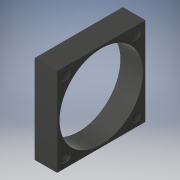
# Autodesk Inventor part: Pi Fan
Saved by Autodesk Inventor 2019 (Build 230136000, 136)
## iProperties
Created: 2018-04-04
Part Number: Pi Fan
Material: PPS Plastic
Document SubType Name: Modeling
Designer: Nikolas X Gamarra
Density: 1.637 g/cm^3
Appearance: Smooth - White(1)
Author: Nikolas X Gamarra
Autodesk Inventor part; units mm, degrees
ref_plane "YZ Plane" through (0, 0, 0) normal (1, 0, 0) x (0, 1, 0)
ref_plane "XZ Plane" through (0, 0, 0) normal (0, 1, 0) x (-1, 0, 0)
ref_plane "XY Plane" through (0, 0, 0) normal (0, 0, 1) x (1, 0, 0)
sketch "Sketch1" plane through (0, 0, 0) normal (1, 0, 0) x (0, 1, 0)
  line L0 (0, 0) -> (30, 0)
  line L1 (30, 0) -> (30, -30)
  line L2 (30, -30) -> (0, -30)
  line L3 (0, -30) -> (0, 0)
  dimension "d0" = 30
  dimension "d1" = 30
  constraints: 8 end point, 2 parallel, 1 horizontal, 1 perpendicular
  measures "d0" distance of L1.end L2.end
  measures "d1" distance of L0.end L1.end
extrude "Extrusion1" add sketch "Sketch1" along normal blind 7.62
sketch "Sketch2" plane through (7.62, 0, 0) normal (1, 0, 0) x (0, 0, -1)
  line L0 (0, 30) -> (0, 0) projected
  line L1 (0, 0) -> (30, 0) projected
  line L2 (30, 0) -> (30, 30) projected
  line L3 (30, 30) -> (0, 30) projected
  line L4 (15, 30) -> (15, 0) construction
  line L5 (0, 15) -> (30, 15) construction
  circle A0 centre (15, 15) radius 14.225
  dimension "d4" = 28.45
  constraints: 5 midpoint, 4 end point, 1 centre point
  measures "d4" diameter of A0
extrude "Extrusion2" cut sketch "Sketch2" against normal blind 7.62 contours A0
sketch "Sketch3" plane through (7.62, 0, 0) normal (1, 0, 0) x (0, 0, -1)
  line L0 (0, 30) -> (30, 30) construction
  line L1 (15, 30) -> (15, 0) construction
  line L2 (30, 0) -> (0, 0) construction
  line L3 (0, 0) -> (0, 30) construction
  line L4 (0, 15) -> (29.023, 15) construction
  point P0 (3, 2.84)
  point P1 (3, 27.16)
  point P2 (27, 2.84)
  point P3 (27, 27.16)
  dimension "d15" = 2.84
  constraints: 4 end point, 3 midpoint, 3 symmetric about line, 1 horizontal
  measures "d15" distance from line of L2 point (3, 2.84)
hole "Hole1" at (7.62, 2.84, -3) at (7.62, 27.16, -3) at (7.62, 27.16, -27) at (7.62, 2.84, -27) direction (-1, 0, 0) diameter 3.175 end through all
body "Solid1"
